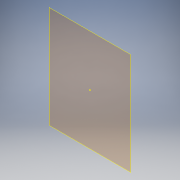
# Autodesk Inventor part: KEEPOUT_TOP_0MM
Saved by Autodesk Inventor 2016 (Build 200138000, 138)
## iProperties
Created: 2016-09-29
Part Number: KEEPOUT_TOP_0MM
Material: Generic
Document SubType Name: Modeling
Designer: benja
Density: 1 g/cm^3
Appearance: Default
Author: benja
Autodesk Inventor part; units mm, degrees
ref_plane "YZ Plane" through (0, 0, 0) normal (1, 0, 0) x (0, 1, 0)
ref_plane "XZ Plane" through (0, 0, 0) normal (0, 1, 0) x (-1, 0, 0)
ref_plane "XY Plane" through (0, 0, 0) normal (0, 0, 1) x (1, 0, 0)
ref_plane "Work Plane1" through (0, 0, 0) normal (0, 0, 1) x (1, 0, 0)
sketch "KEEPOUT_TOP_0.1MM_S" plane through (0, 0, 0) normal (0, 0, 1) x (1, 0, 0)
  circle A0 centre (0, -25) radius 1.75 projected
  circle A1 centre (14, -14) radius 1.75 projected
  circle A2 centre (-22, -14) radius 1.75 projected
  circle A3 centre (-14, 14) radius 1.75 projected
  circle A4 centre (22, 14) radius 1.75 projected
  circle A5 centre (0, 30) radius 1.75 projected
  line L0 (30, 22.5) -> (30, -22.5) projected
  arc A6 (30, 22.5) -> (-30, 22.5) centre (0, 0) ccw projected
  line L1 (-30, -22.5) -> (-30, 22.5) projected
  arc A7 (-30, -22.5) -> (30, -22.5) centre (0, 0) ccw projected
  line L2 (29.5, -22.3327) -> (29.5, 22.3327)
  arc A8 (29.5, 22.3327) -> (-29.5, 22.3327) centre (0, 0) ccw
  line L3 (-29.5, 22.3327) -> (-29.5, -22.3327)
  arc A9 (-29.5, -22.3327) -> (29.5, -22.3327) centre (0, 0) ccw
  line L4 (18.25, -29.3526) -> (18.25, -17.75) projected
  line L5 (25.75, -20.8034) -> (25.75, -23.3524) projected
  line L6 (18.75, -24) -> (26.1582, -24) projected
  line L7 (-9, 11) -> (-9, 17) projected
  line L8 (-17, 10) -> (-10, 10) projected
  line L9 (-18.25, 10.25) -> (-18.25, -10.25) projected
  line L10 (-25, -18) -> (-19, -18) projected
  line L11 (-18, -17) -> (-18, 9) projected
  line L12 (18, 17) -> (18, -9) projected
  line L13 (17, -10) -> (10, -10) projected
  line L14 (9, -11) -> (9, -17) projected
  line L15 (10, -18) -> (25, -18) projected
  line L16 (27, -18) -> (35.3377, -18) projected
  line L17 (33, -7.9807) -> (27, -7.9807) projected
  line L18 (27, 7.9807) -> (33, 7.9807) projected
  line L19 (35.3377, 18) -> (27, 18) projected
  line L20 (29.5, 18.5) -> (17.5, 18.5)
  line L21 (17.5, 18.5) -> (17.5, -9.5)
  line L22 (17.5, -9.5) -> (8.5, -9.5)
  line L23 (8.5, -9.5) -> (8.5, -18.5)
  line L24 (8.5, -18.5) -> (29.5, -18.5)
  line L25 (29.5, -7.4807) -> (27.05, -7.4807)
  line L26 (27.05, -7.4807) -> (27.05, 7.4807)
  line L27 (27.05, 7.4807) -> (29.5, 7.4807)
  line L28 (29.5, 7.4807) -> (29.5, -7.4807)
  circle A10 centre (0, -25) radius 3.5
  circle A11 centre (0, 30) radius 3.5
  line L29 (-29.5, -18.5) -> (-17.5, -18.5)
  line L30 (-17.5, -18.5) -> (-17.5, 9.5)
  line L31 (-17.5, 9.5) -> (-8.5, 9.5)
  line L32 (-8.5, 9.5) -> (-8.5, 18.5)
  line L33 (-8.5, 18.5) -> (-29.5, 18.5)
  line L34 (-29.5, -7.4807) -> (-27.05, -7.4807)
  line L35 (-27.05, -7.4807) -> (-27.05, 7.4807)
  line L36 (-27.05, 7.4807) -> (-29.5, 7.4807)
  line L37 (-29.5, 7.4807) -> (-29.5, -7.4807)
  line L38 (-6.5943, -38.4385) -> (-6.1249, -35.4751) projected
  arc A12 (-33.4813, -20) -> (-6.5943, -38.4385) centre (0, 0) ccw projected
  line L39 (-29.5931, -20) -> (-33.4813, -20) projected
  arc A13 (-29.1821, -20.2153) -> (-29.5931, -20) centre (-29.5931, -20.5) ccw projected
  arc A14 (-29.1821, -20.2153) -> (-25.6905, -24.5) centre (0, 0) ccw projected
  line L40 (-18.75, -24.5) -> (-25.6905, -24.5) projected
  line L41 (-18.75, -29.2948) -> (-18.75, -24.5) projected
  arc A15 (-18.75, -29.2948) -> (-17.4627, -31.481) centre (-16.25, -29.2948) ccw projected
  arc A16 (-17.4627, -31.481) -> (-6.1249, -35.4751) centre (0, 0) ccw projected
  line L42 (26.1751, -24.5) -> (18.75, -24.5) projected
  spline S0 degree 3 poles (26.25, -24.6361) (26.2495, -24.6351) (26.2489, -24.6341) (26.225, -24.5909) (26.2003, -24.5462) (26.1751, -24.5) knots -0.000336 -0.000336 -0.000336 -0.000336 0 0 0.014472 0.014472 0.014472 0.014472 projected
  arc A17 (26.25, -24.6361) -> (29.9333, -20) centre (0, 0) ccw projected
  line L43 (29.9333, -20) -> (33.4813, -20) projected
  arc A18 (6.5943, -38.4385) -> (33.4813, -20) centre (0, 0) ccw projected
  line L44 (6.1249, -35.4751) -> (6.5943, -38.4385) projected
  arc A19 (6.1249, -35.4751) -> (17.4627, -31.481) centre (0, 0) ccw projected
  arc A20 (17.4627, -31.481) -> (18.75, -29.2948) centre (16.25, -29.2948) ccw projected
  line L45 (18.75, -24.5) -> (18.75, -29.2948) projected
  line L46 (-18.25, -17.75) -> (-18.25, -29.3526) projected
  line L47 (-26.1582, -24) -> (-18.75, -24) projected
  arc A21 (-17.2201, -31.0438) -> (-7.4928, -34.7003) centre (0, 0) ccw projected
  arc A22 (7.4928, -34.7003) -> (17.2201, -31.0438) centre (0, 0) ccw projected
  line L48 (5.6311, -35.5534) -> (6.2569, -39.5044) projected
  line L49 (-6.2569, -39.5044) -> (-5.6311, -35.5534) projected
  arc A23 (26.3818, -23) -> (29.5, -18.8348) centre (0, 0) ccw
  line L50 (26.3818, -23) -> (17.75, -23)
  line L51 (17.75, -23) -> (17.75, -30.1652)
  arc A24 (4.9808, -34.6438) -> (17.75, -30.1652) centre (0, 0) ccw
  line L52 (4.9808, -34.6438) -> (5.2937, -36.6193)
  arc A25 (-17.75, -30.1652) -> (-4.9808, -34.6438) centre (0, 0) ccw
  line L53 (-17.75, -30.1652) -> (-17.75, -23)
  line L54 (-17.75, -23) -> (-26.3818, -23)
  arc A26 (-29.5, -18.8348) -> (-26.3818, -23) centre (0, 0) ccw
  line L55 (-5.6311, 35.5534) -> (-6.2569, 39.5044) projected
  arc A27 (-7.4928, 34.7003) -> (-17.2201, 31.0438) centre (0, 0) ccw projected
  line L56 (-18.25, 29.3526) -> (-18.25, 17.75) projected
  line L57 (-18.75, 24) -> (-26.1582, 24) projected
  arc A28 (-26.625, 23.481) -> (-28.0998, 21.6944) centre (0, 0) ccw projected
  arc A29 (-25.9374, 23.5) -> (-29.5, 18.8348) centre (0, 0) ccw
  line L58 (-25.9374, 23.5) -> (-17.75, 23.5)
  line L59 (-17.75, 23.5) -> (-17.75, 30.1652)
  arc A30 (-4.9808, 34.6438) -> (-17.75, 30.1652) centre (0, 0) ccw
  arc A31 (17.75, 30.1652) -> (4.9808, 34.6438) centre (0, 0) ccw
  line L60 (26.1582, 24) -> (18.75, 24) projected
  line L61 (18.25, 17.75) -> (18.25, 29.3526) projected
  arc A32 (28.0998, 21.6944) -> (26.625, 23.481) centre (0, 0) ccw projected
  line L62 (17.75, 30.1652) -> (17.75, 23.5)
  line L63 (17.75, 23.5) -> (25.9374, 23.5)
  arc A33 (29.5, 18.8348) -> (25.9374, 23.5) centre (0, 0) ccw
  line L64 (4.9808, 34.6438) -> (5.2937, 36.6193)
  line L65 (-4.9808, -34.6438) -> (-5.2937, -36.6193)
  line L66 (-10, 18) -> (-25, 18) projected
  arc A34 (17.2201, 31.0438) -> (7.4928, 34.7003) centre (0, 0) ccw projected
  line L67 (6.2569, 39.5044) -> (5.6311, 35.5534) projected
  line L68 (27, 18) -> (25, 18) projected
  line L69 (18, 17) -> (18, -9) projected
  arc A35 (-26, 17) -> (-27, 18) centre (-27, 17) ccw projected
  line L70 (-27, 18) -> (-35.3377, 18) projected
  arc A36 (-35.3377, 18) -> (-36.6968, 17.1346) centre (-35.3377, 16.5) ccw projected
  arc A37 (-36.6968, 17.1346) -> (-36.6968, -17.1346) centre (0, 0) ccw projected
  arc A38 (-36.6968, -17.1346) -> (-35.3377, -18) centre (-35.3377, -16.5) ccw projected
  line L71 (-35.3377, -18) -> (-27, -18) projected
  arc A39 (-27, -18) -> (-26, -17) centre (-27, -17) ccw projected
  line L72 (-26, -17) -> (-26, -8.9807) projected
  arc A40 (-26, -8.9807) -> (-27, -7.9807) centre (-27, -8.9807) ccw projected
  line L73 (-27, -7.9807) -> (-33, -7.9807) projected
  arc A41 (-34, -6.9807) -> (-33, -7.9807) centre (-33, -6.9807) ccw projected
  line L74 (-34, -6.9807) -> (-34, 6.9807) projected
  arc A42 (-33, 7.9807) -> (-34, 6.9807) centre (-33, 6.9807) ccw projected
  line L75 (-33, 7.9807) -> (-27, 7.9807) projected
  arc A43 (-27, 7.9807) -> (-26, 8.9807) centre (-27, 8.9807) ccw projected
  line L76 (-26, 8.9807) -> (-26, 17) projected
  circle A44 centre (-30, 14.5) radius 1.75 projected
  circle A45 centre (-30, -14.5) radius 1.75 projected
  line L77 (-26.55, -15.6278) -> (-26.55, 4.9922) projected
  line L78 (-27.4, -5) -> (-27.4, 5) projected
  line L79 (-26.55, -15.6278) -> (-26.55, 4.9922) projected
  line L80 (26.55, 15.6278) -> (26.55, -4.9922) projected
  line L81 (-4.9808, 34.6438) -> (-5.2937, 36.6193)
  line L82 (-29.5, 18.8348) -> (-29.5, 22.3327)
  point P0 (0, 0)
  dimension "d0" = 0.5
  dimension "d1" = 7
  dimension "d2" = 7
  dimension "d3" = 1
  dimension "d4" = 1
  dimension "d5" = 0.5
  dimension "d6" = 0.5
  dimension "d7" = 0.5
  dimension "d8" = 0.5
  dimension "d9" = 0.5
  dimension "d10" = 0.5
  dimension "d11" = 1
  dimension "d12" = 0.5
  dimension "d13" = 0.5
  dimension "d14" = 0.5
  dimension "d15" = 0.5
  dimension "d16" = 0.5
  dimension "d17" = 0.5
  dimension "d18" = 0.5
  dimension "d19" = 0.5
  dimension "d20" = 0.5
  dimension "d21" = 0.5
  dimension "d23" = 0.5
  dimension "d24" = 0.5
  dimension "d25" = 0.5
  dimension "d26" = 0.5
  dimension "d27" = 0.5
  dimension "d28" = 0.5
  dimension "d29" = 0.5
  dimension "d30" = 0.5
  dimension "d31" = 0.5
  dimension "d32" = 0.5
  dimension "d33" = 0.5
  dimension "d34" = 0.5
  dimension "d35" = 0.5
  dimension "d36" = 0.5
  dimension "d37" = 0.5
  dimension "d38" = 0.5
  constraints: 67 end point, 24 point on circle, 13 perpendicular, 12 centre point, 10 coincident, 10 point on line, 9 parallel, 5 horizontal, 2 vertical, 1 collinear, 3 other
  measures "d0" radial gap between concentric circles of A7 A9
  measures "d1" diameter of A10
  measures "d2" diameter of A11
  measures "d3" radial gap between concentric circles of A23 A17
  measures "d4" distance between parallel lines of L6 L50
  measures "d5" distance between parallel lines of L4 L51
  measures "d6" radial gap between concentric circles of A22 A24
  measures "d7" distance between parallel lines of L48 L52
  measures "d8" distance between parallel lines of L49 L65
  measures "d9" radial gap between concentric circles of A21 A25
  measures "d10" distance between parallel lines of L46 L53
  measures "d11" distance between parallel lines of L47 L54
  measures "d12" radial gap between concentric circles of A14 A26
  measures "d13" distance between parallel lines of L29 L10
  measures "d14" distance between parallel lines of L11 L30
  measures "d15" distance between parallel lines of L8 L31
  measures "d16" distance between parallel lines of L7 L32
  measures "d17" distance between parallel lines of L66 L33
  measures "d18" radial gap between concentric circles of A28 A29
  measures "d19" distance between parallel lines of L57 L58
  measures "d20" distance between parallel lines of L56 L59
  measures "d21" radial gap between concentric circles of A27 A30
  measures "d23" distance between parallel lines of L64 L67
  measures "d24" radial gap between concentric circles of A31 A34
  measures "d25" distance between parallel lines of L62 L61
  measures "d26" distance between parallel lines of L60 L63
  measures "d27" radial gap between concentric circles of A32 A33
  measures "d28" distance between parallel lines of L68 L20
  measures "d29" distance between parallel lines of L12 L21
  measures "d30" distance between parallel lines of L13 L22
  measures "d31" distance between parallel lines of L23 L14
  measures "d32" distance between parallel lines of L24 L15
  measures "d33" distance between parallel lines of L77 L35
  measures "d34" distance between parallel lines of L73 L34
  measures "d35" distance between parallel lines of L75 L36
  measures "d36" distance between parallel lines of L17 L25
  measures "d37" distance between parallel lines of L80 L26
  measures "d38" distance between parallel lines of L18 L27
extrude "KEEPOUT_TOP_0.1MM" add sketch "KEEPOUT_TOP_0.1MM_S" along normal blind 0.1 contours A0 | A1 | A2 | A3 | A4 | A5 | L0 L19 L2 A8 L67 A6 | L0 L18 L2 L19 | L67 A8 L55 A6 | L0 L17 L2 L18 | L2 L27 L26 L25 L24 L23 L22 L21 L20 | L55 A8 L3 L70 L1 A6 | A8 L2 A33 L63 L62 A31 L64 | L0 L16 L2 L17 | A8 L81 A30 L59 L58 A29 L3 | L0 L43 A17 L2 L16 | L70 L3 A44 L1 | L0 A7 L44 A9 L2 A17 L43 | A44 L3 L1 | L70 A35 L76 A43 L75 L3 A44 | L3 L33 L32 L31 L30 L29 L71 A39 L72 A40 L73 L34 L35 L36 L75 A43 L76 A35 L70 | A44 L3 L75 L1 | A44 L3 | A7 L48 A9 L44 | A17 S0 L42 L45 A20 A19 L44 A9 L52 A24 L51 L50 A23 L2 | L2 A9 L44 A19 A20 L45 L42 S0 A17 | L75 L3 L73 L1 | A7 L49 A9 L48 | L73 L3 A45 L1 | A7 L38 A9 L49 | A45 L3 L1 | L73 A40 L72 A39 L71 L3 A45 | L36 L35 L34 L3 | L71 L3 A13 L39 L1 | L1 A45 L3 L71 | A7 L1 L39 A13 L3 A9 L38 | A9 L38 A16 A15 L41 L40 A14 A13 L3 A26 L54 L53 A25 L65 | A45 L3 | A9 L3 A13 A14 L40 L41 A15 A16 L38 | A10 | A11
ref_plane "Work Plane2" through (0, 0, 0) normal (0, 0, 1) x (1, 0, 0)
sketch "KEEPOUT_TOP_5MM_S" plane through (0, 0, 0) normal (0, 0, 1) x (1, 0, 0)
  line L0 (-29.5, 7.4807) -> (-27.05, 7.4807) projected
  line L1 (-27.05, 7.4807) -> (-27.05, -7.4807) projected
  line L2 (-27.05, -7.4807) -> (-29.5, -7.4807) projected
  line L3 (-29.5, -7.4807) -> (-29.5, 7.4807) projected
  line L4 (30, -22.5) -> (30, 22.5) projected
  arc A0 (30, 22.5) -> (-30, 22.5) centre (0, 0) ccw projected
  line L5 (-30, 22.5) -> (-30, -22.5) projected
  arc A1 (-30, -22.5) -> (30, -22.5) centre (0, 0) ccw projected
  line L6 (29.5, -7.4807) -> (27.05, -7.4807) projected
  line L7 (27.05, -7.4807) -> (27.05, 7.4807) projected
  line L8 (27.05, 7.4807) -> (29.5, 7.4807) projected
  line L9 (29.5, 7.4807) -> (29.5, -7.4807) projected
  line L10 (-29.5, 18.5) -> (-29.5, 18.8348) projected
  arc A2 (-25.9374, 23.5) -> (-29.5, 18.8348) centre (0, 0) ccw projected
  line L11 (-25.9374, 23.5) -> (-17.75, 23.5) projected
  line L12 (-17.75, 23.5) -> (-17.75, 30.1652) projected
  arc A3 (-4.9808, 34.6438) -> (-17.75, 30.1652) centre (0, 0) ccw projected
  line L13 (-4.9808, 34.6438) -> (-5.2937, 36.6193) projected
  arc A4 (5.2937, 36.6193) -> (-5.2937, 36.6193) centre (0, 0) ccw projected
  line L14 (5.2937, 36.6193) -> (4.9808, 34.6438) projected
  arc A5 (17.75, 30.1652) -> (4.9808, 34.6438) centre (0, 0) ccw projected
  line L15 (17.75, 30.1652) -> (17.75, 23.5) projected
  line L16 (17.75, 23.5) -> (25.9374, 23.5) projected
  arc A6 (29.5, 18.8348) -> (25.9374, 23.5) centre (0, 0) ccw projected
  line L17 (29.5, 18.8348) -> (29.5, 18.5) projected
  line L18 (29.5, 18.5) -> (17.5, 18.5) projected
  line L19 (17.5, 18.5) -> (17.5, -9.5) projected
  line L20 (17.5, -9.5) -> (8.5, -9.5) projected
  line L21 (8.5, -9.5) -> (8.5, -18.5) projected
  line L22 (8.5, -18.5) -> (29.5, -18.5) projected
  line L23 (29.5, -18.5) -> (29.5, -18.8348) projected
  arc A7 (26.3818, -23) -> (29.5, -18.8348) centre (0, 0) ccw projected
  line L24 (26.3818, -23) -> (17.75, -23) projected
  line L25 (17.75, -23) -> (17.75, -30.1652) projected
  arc A8 (4.9808, -34.6438) -> (17.75, -30.1652) centre (0, 0) ccw projected
  line L26 (4.9808, -34.6438) -> (5.2937, -36.6193) projected
  arc A9 (-5.2937, -36.6193) -> (5.2937, -36.6193) centre (0, 0) ccw projected
  line L27 (-5.2937, -36.6193) -> (-4.9808, -34.6438) projected
  arc A10 (-17.75, -30.1652) -> (-4.9808, -34.6438) centre (0, 0) ccw projected
  line L28 (-17.75, -30.1652) -> (-17.75, -23) projected
  line L29 (-17.75, -23) -> (-26.3818, -23) projected
  arc A11 (-29.5, -18.8348) -> (-26.3818, -23) centre (0, 0) ccw projected
  line L30 (-29.5, -18.8348) -> (-29.5, -18.5) projected
  line L31 (-29.5, -18.5) -> (-17.5, -18.5) projected
  line L32 (-17.5, -18.5) -> (-17.5, 9.5) projected
  line L33 (-17.5, 9.5) -> (-8.5, 9.5) projected
  line L34 (-8.5, 9.5) -> (-8.5, 18.5) projected
  line L35 (-8.5, 18.5) -> (-29.5, 18.5) projected
  line L36 (25.75, -20.8034) -> (25.75, -23.3524) projected
  line L37 (18.25, -29.3526) -> (18.25, -17.75) projected
  line L38 (-18.25, -17.75) -> (-18.25, -29.3526) projected
  line L39 (-25.75, -23.3524) -> (-25.75, -20.8034) projected
  line L40 (18.25, 17.75) -> (18.25, 29.3526) projected
  line L41 (25.75, 23.3524) -> (25.75, 20.8034) projected
  line L42 (-18.25, 29.3526) -> (-18.25, 17.75) projected
  line L43 (-25.75, 20.8034) -> (-25.75, 23.3524) projected
  line L44 (17.75, 23.5) -> (17.75, 18.5)
  line L45 (29.5, 18.5) -> (17.5, 18.5) projected
  line L46 (26.25, 18.5) -> (26.25, 23.1503)
  arc A12 (29.5, 18.8348) -> (25.9374, 23.5) centre (0, 0) ccw projected
  line L47 (17.75, -23) -> (17.75, -18.5)
  line L48 (8.5, -18.5) -> (29.5, -18.5) projected
  line L49 (26.3818, -23) -> (17.75, -23) projected
  line L50 (26.25, -23) -> (26.25, -18.5)
  line L51 (-26.3818, -23) -> (-17.75, -23) projected
  line L52 (-17.75, -23) -> (-17.75, -18.5)
  line L53 (-29.5, -18.5) -> (-17.5, -18.5) projected
  line L54 (-26.25, -18.5) -> (-26.25, -23.1503)
  arc A13 (-29.5, -18.8348) -> (-26.3818, -23) centre (0, 0) ccw projected
  arc A14 (26.25, 23.1503) -> (25.9374, 23.5) centre (0, 0) ccw
  arc A15 (29.5, 18.8348) -> (25.9374, 23.5) centre (0, 0) ccw projected
  line L55 (26.25, 18.5) -> (17.75, 18.5)
  line L56 (17.75, 23.5) -> (25.9374, 23.5)
  line L57 (26.25, -23) -> (17.75, -23)
  line L58 (26.25, -18.5) -> (17.75, -18.5)
  line L59 (-25.9374, 23.5) -> (-17.75, 23.5) projected
  line L60 (-17.75, 23.5) -> (-17.75, 18.5)
  line L61 (-17.75, 18.5) -> (-26.25, 18.5)
  line L62 (-29.5, 18.5) -> (-8.5, 18.5) projected
  line L63 (-26.25, 18.5) -> (-26.25, 23.1503)
  arc A16 (-25.9374, 23.5) -> (-29.5, 18.8348) centre (0, 0) ccw projected
  arc A17 (-25.9374, 23.5) -> (-26.25, 23.1503) centre (0, 0) ccw
  line L64 (-25.9374, 23.5) -> (-17.75, 23.5)
  line L65 (-17.75, -23) -> (-26.25, -23)
  line L66 (-17.75, -18.5) -> (-26.25, -18.5)
  line L67 (-17.75, 23.5) -> (-25.9374, 23.5)
  line L68 (26.25, 18.5) -> (17.75, 18.5)
  point P0 (0, 0)
  dimension "d43" = 0.5
  dimension "d44" = 0.5
  dimension "d45" = 0.5
  dimension "d46" = 0.5
  constraints: 36 end point, 11 point on line, 9 point on circle, 7 perpendicular, 5 parallel, 3 collinear, 2 centre point, 2 concentric, 1 horizontal
  measures "d43" distance between parallel lines of L41 L46
  measures "d44" distance between parallel lines of L36 L50
  measures "d45" distance between parallel lines of L39 L54
  measures "d46" distance between parallel lines of L63 L43
extrude "KEEPOUT_TOP_5MM" add sketch "KEEPOUT_TOP_5MM_S" along normal blind 5 contours L63 A2 L11 L42 L35 | L42 L11 L60 L35 | L52 L29 L38 L31 | L38 L29 L54 L31 | L16 L40 L18 L44 | L16 A6 L46 L18 L40 | L47 L22 L37 L24 | L37 L22 L50 L24
ref_plane "Work Plane3" through (0, 0, 0) normal (0, 0, 1) x (1, 0, 0)
sketch "KEEPOUT_TOP_9.5MM_S" plane through (0, 0, 0) normal (0, 0, 1) x (1, 0, 0)
  line L0 (-29.5, 7.4807) -> (-27.05, 7.4807)
  line L1 (-27.05, 7.4807) -> (-27.05, -7.4807)
  line L2 (-27.05, -7.4807) -> (-29.5, -7.4807)
  line L3 (-29.5, -7.4807) -> (-29.5, 7.4807)
  line L4 (30, -22.5) -> (30, 22.5)
  arc A0 (30, 22.5) -> (-30, 22.5) centre (0, 0) ccw
  line L5 (-30, 22.5) -> (-30, -22.5)
  arc A1 (-30, -22.5) -> (30, -22.5) centre (0, 0) ccw
  line L6 (29.5, -7.4807) -> (27.05, -7.4807)
  line L7 (27.05, -7.4807) -> (27.05, 7.4807)
  line L8 (27.05, 7.4807) -> (29.5, 7.4807)
  line L9 (29.5, 7.4807) -> (29.5, -7.4807)
  line L10 (-29.5, 18.5) -> (-29.5, 18.8348)
  arc A2 (-26.25, 23.1503) -> (-29.5, 18.8348) centre (0, 0) ccw
  arc A3 (-25.9374, 23.5) -> (-26.25, 23.1503) centre (0, 0) ccw
  line L11 (-25.9374, 23.5) -> (-17.75, 23.5)
  line L12 (-17.75, 23.5) -> (-17.75, 30.1652)
  arc A4 (-4.9808, 34.6438) -> (-17.75, 30.1652) centre (0, 0) ccw
  line L13 (-4.9808, 34.6438) -> (-5.2937, 36.6193)
  arc A5 (5.2937, 36.6193) -> (-5.2937, 36.6193) centre (0, 0) ccw
  line L14 (5.2937, 36.6193) -> (4.9808, 34.6438)
  arc A6 (17.75, 30.1652) -> (4.9808, 34.6438) centre (0, 0) ccw
  line L15 (17.75, 30.1652) -> (17.75, 23.5)
  line L16 (17.75, 23.5) -> (25.9374, 23.5)
  arc A7 (26.25, 23.1503) -> (25.9374, 23.5) centre (0, 0) ccw
  arc A8 (29.5, 18.8348) -> (26.25, 23.1503) centre (0, 0) ccw
  line L17 (29.5, 18.8348) -> (29.5, 18.5)
  line L18 (29.5, 18.5) -> (26.25, 18.5)
  line L19 (26.25, 18.5) -> (17.75, 18.5)
  line L20 (17.75, 18.5) -> (17.5, 18.5)
  line L21 (17.5, 18.5) -> (17.5, -9.5)
  line L22 (17.5, -9.5) -> (8.5, -9.5)
  line L23 (8.5, -9.5) -> (8.5, -18.5)
  line L24 (8.5, -18.5) -> (17.75, -18.5)
  line L25 (17.75, -18.5) -> (26.25, -18.5)
  line L26 (26.25, -18.5) -> (29.5, -18.5)
  line L27 (29.5, -18.5) -> (29.5, -18.8348)
  arc A9 (26.3818, -23) -> (29.5, -18.8348) centre (0, 0) ccw
  line L28 (26.3818, -23) -> (26.25, -23)
  line L29 (26.25, -23) -> (17.75, -23)
  line L30 (17.75, -23) -> (17.75, -30.1652)
  arc A10 (4.9808, -34.6438) -> (17.75, -30.1652) centre (0, 0) ccw
  line L31 (4.9808, -34.6438) -> (5.2937, -36.6193)
  arc A11 (-5.2937, -36.6193) -> (5.2937, -36.6193) centre (0, 0) ccw
  line L32 (-5.2937, -36.6193) -> (-4.9808, -34.6438)
  arc A12 (-17.75, -30.1652) -> (-4.9808, -34.6438) centre (0, 0) ccw
  line L33 (-17.75, -30.1652) -> (-17.75, -23)
  line L34 (-17.75, -23) -> (-26.25, -23)
  line L35 (-26.25, -23) -> (-26.3818, -23)
  arc A13 (-29.5, -18.8348) -> (-26.3818, -23) centre (0, 0) ccw
  line L36 (-29.5, -18.8348) -> (-29.5, -18.5)
  line L37 (-29.5, -18.5) -> (-26.25, -18.5)
  line L38 (-26.25, -18.5) -> (-17.75, -18.5)
  line L39 (-17.75, -18.5) -> (-17.5, -18.5)
  line L40 (-17.5, -18.5) -> (-17.5, 9.5)
  line L41 (-17.5, 9.5) -> (-8.5, 9.5)
  line L42 (-8.5, 9.5) -> (-8.5, 18.5)
  line L43 (-8.5, 18.5) -> (-17.75, 18.5)
  line L44 (-17.75, 18.5) -> (-26.25, 18.5)
  line L45 (-26.25, 18.5) -> (-29.5, 18.5)
  line L46 (17.75, 23.5) -> (17.75, 18.5)
  line L47 (17.75, 18.5) -> (26.25, 18.5)
  line L48 (26.25, 18.5) -> (26.25, 23.1503)
  arc A14 (26.25, 23.1503) -> (25.9374, 23.5) centre (0, 0) ccw
  line L49 (25.9374, 23.5) -> (17.75, 23.5)
  line L50 (26.25, -23) -> (26.25, -18.5)
  line L51 (26.25, -18.5) -> (17.75, -18.5)
  line L52 (17.75, -18.5) -> (17.75, -23)
  line L53 (17.75, -23) -> (26.25, -23)
  line L54 (-17.75, -23) -> (-17.75, -18.5)
  line L55 (-17.75, -18.5) -> (-26.25, -18.5)
  line L56 (-26.25, -18.5) -> (-26.25, -23)
  line L57 (-26.25, -23) -> (-17.75, -23)
  line L58 (-17.75, 18.5) -> (-17.75, 23.5)
  line L59 (-26.25, 23.1503) -> (-26.25, 18.5)
  line L60 (-26.25, 18.5) -> (-17.75, 18.5)
  line L61 (-17.75, 18.5) -> (-17.75, 23.5)
  line L62 (-17.75, 23.5) -> (-25.9374, 23.5)
  arc A15 (-25.9374, 23.5) -> (-26.25, 23.1503) centre (0, 0) ccw
  circle A16 centre (0, 30) radius 3.5
  circle A17 centre (0, -25) radius 3.465
  point P0 (0, 0)
extrude "KEEPOUT_TOP_9.5MM" add sketch "KEEPOUT_TOP_9.5MM_S" along normal blind 9.5 separate body contours L0 L1 L2 L3 | L6 L7 L8 L9 | L10 A2 L59 L45 | L58 L12 A4 L13 A5 L14 A6 L15 L46 L20 L21 L22 L23 L24 L52 L30 A10 L31 A11 L32 A12 L33 L54 L39 L40 L41 L42 L43 | L56 L35 A13 L36 L37 | A8 L17 L18 L48 | L50 L26 L27 A9 L28
equation "\"d7\" = d6"
equation "\"d8\" = d7"
equation "\"d9\" = d8"
equation "\"d10\" = d9"
equation "\"d12\" = d10"
equation "\"d13\" = d12"
equation "\"d14\" = d13"
equation "\"d15\" = d14"
equation "\"d16\" = d15"
equation "\"d17\" = d16"
equation "\"d18\" = d17"
equation "\"d19\" = d17"
equation "\"d20\" = d19"
equation "\"d21\" = d20"
equation "\"d24\" = d23"
equation "\"d25\" = d24"
equation "\"d26\" = d25"
equation "\"d27\" = d26"
equation "\"d28\" = d26"
equation "\"d29\" = d28"
equation "\"d30\" = d29"
equation "\"d31\" = d30"
equation "\"d32\" = d31"
equation "\"d33\" = d14"
equation "\"d34\" = d14"
equation "\"d35\" = d33"
equation "\"d36\" = d30"
equation "\"d37\" = d28"
equation "\"d38\" = d36"
body "Solid2"
body "Solid3"
